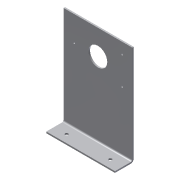
# Autodesk Inventor part: Part154
Saved by Autodesk Inventor 2014 SP2 (Build 180246200, 246)
## iProperties
Created: 2014-12-15
Part Number: Part154
Material: Aluminum 6061
Document SubType Name: Sheet Metal
Designer: Admin
Density: 2.71 g/cm^3
Sheet Metal Rule: Default
Appearance: Aluminum - Flat
Author: Admin
Autodesk Inventor part; units mm, degrees
ref_plane "YZ Plane" through (0, 0, 0) normal (1, 0, 0) x (0, 1, 0)
ref_plane "XZ Plane" through (0, 0, 0) normal (0, 1, 0) x (-1, 0, 0)
ref_plane "XY Plane" through (0, 0, 0) normal (0, 0, 1) x (1, 0, 0)
sketch "Sketch1" plane through (0, 0, 0) normal (0, 0, 1) x (1, 0, 0)
  line L0 (0, 0) -> (139.7, 0)
  line L1 (139.7, 0) -> (139.7, 203.2)
  line L2 (139.7, 203.2) -> (0, 203.2)
  line L3 (0, 203.2) -> (0, 0)
  dimension "d0" = 139.7
  dimension "d1" = 203.2
  measures "d0" distance of L2.end L1.end
  measures "d1" distance of L1.end L0.end
extrude "Plate1" add sketch "Sketch1" along normal blind 3.048
sketch "Sketch2" plane through (139.7, 3.048, 0) normal (0, -1, 0) x (1, 0, 0)
  line L0 (-139.7, 0) -> (0, 0)
  line L1 (0, 0) -> (0, 38.1)
  line L2 (0, 38.1) -> (-139.7, 38.1)
  line L3 (-139.7, 38.1) -> (-139.7, 0)
  constraints: 6 end point, 1 horizontal, 1 perpendicular, 1 vertical
edge flange "Flange1" height 38.1 angle 90 thickness 3.048 bend radius 3.048 thickness toward (0, -1, 0) relief tear relief width 3.048 relief depth 1.524 edges at (69.85, 0, 3.048) wall of the first edge with corners at (0, 3.048, 0) (139.7, 3.048, 0) (139.7, 3.048, 38.1) (0, 3.048, 38.1)
bend "Bend1"
corner "Corner1"
sketch "Sketch3" plane through (0, 0, 3.048) normal (0, 0, 1) x (1, 0, 0)
  line L0 (139.7, 203.2) -> (139.7, 6.096) projected
  line L1 (0, 203.2) -> (139.7, 203.2) projected
  circle A0 centre (21.4376, 152.4) radius 2.0638
  circle A1 centre (118.8466, 124.1044) radius 2.0638
  circle A2 centre (118.6688, 180.9242) radius 2.0637
  point P0 (0, 0)
  dimension "d13" = 20.8534
  dimension "d14" = 79.0956
  dimension "d16" = 21.0312
  dimension "d18" = 50.8
  dimension "d19" = 22.2758
  dimension "d20" = 4.1275
  dimension "d21" = 4.1275
  dimension "d22" = 4.1275
  dimension "d39" = 118.2624
  constraints: 3 centre point, 3 coincident
  measures "d13" distance from line of L0 point (118.847, 124.104)
  measures "d14" distance from line of L1 point (118.847, 124.104)
  measures "d16" distance from line of point (118.669, 180.924) L0
  measures "d18" distance from line of L1 point (21.438, 152.4)
  measures "d19" distance from line of L1 point (118.669, 180.924)
  measures "d20" diameter of A0
  measures "d21" diameter of A1
  measures "d22" diameter of A2
  measures "d39" distance from line of L0 point (21.438, 152.4)
hole "Hole1" at (118.8466, 124.1044, 3.048) at (118.6688, 180.9242, 3.048) at (21.4376, 152.4, 3.048) direction (0, 0, -1) diameter 4.1275 end through all
sketch "Sketch4" plane through (0, 3.048, 38.1) normal (0, 1, 0) x (1, 0, 0)
  line L0 (0, 0) -> (0, 32.004) projected
  line L1 (139.7, 0) -> (139.7, 32.004) projected
  point P0 (0, 38.1)
  point P1 (25.4, 16.002)
  point P2 (114.3, 16.002)
  dimension "d30" = 25.4
  dimension "d31" = 25.4
  measures "d30" distance from line of point (25.4, 16.002) L0
  measures "d31" distance from line of L1 point (114.3, 16.002)
hole "Hole2" at (25.4, 3.048, 22.098) at (114.3, 3.048, 22.098) direction (0, -1, 0) diameter 6.35 end through all
sketch "Sketch5" plane through (0, 0, 3.048) normal (0, 0, 1) x (1, 0, 0)
  line L0 (139.7, 203.2) -> (139.7, 6.096) projected
  line L1 (0, 203.2) -> (139.7, 203.2) projected
  point P0 (0, 0)
  point P1 (69.85, 152.4)
  dimension "d40" = 50.8
  dimension "d41" = 69.85
  measures "d40" distance from line of L1 point (69.85, 152.4)
  measures "d41" distance from line of L0 point (69.85, 152.4)
hole "Hole3" at (69.85, 152.4, 3.048) direction (0, 0, -1) diameter 38.1 end through all
equation "\"d28\" = Thickness"
equation "\"d37\" = Thickness"
equation "\"d47\" = Thickness"
equation "\"d3\" = BendReliefWidth"
equation "\"d4\" = BendReliefDepth"
equation "\"d5\" = MinimumRemnant"
equation "\"d6\" = BendRadius"
equation "\"d9\" = BendRadius"
equation "\"d10\" = CornerReliefSize"
equation "\"d11\" = GapSize"
equation "\"d12\" = JacobiRadiusSize"
equation "\"BendRadius\" = Thickness"
equation "\"BendReliefWidth\" = Thickness"
equation "\"BendReliefDepth\" = 0.5 * Thickness"
equation "\"CornerReliefSize\" = 4 * Thickness"
equation "\"MinimumRemnant\" = 2 * Thickness"
equation "\"TransitionRadius\" = BendRadius"
equation "\"JacobiRadiusSize\" = BendRadius"
equation "\"GapSize\" = Thickness"
equation "\"d2\" = BendRadius"
equation "\"Thickness\" = 3.048"
body "Solid1"
